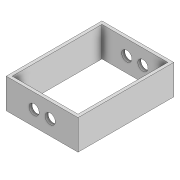
# Autodesk Inventor part: 본체 겉면
Saved by Autodesk Inventor 2020 (Build 240168000, 168)
## iProperties
Created: 2022-08-24
Part Number: 본체 겉면
Material: 일반
Document SubType Name: Modeling
Designer: 박연호
Density: 1 g/cm^3
Appearance: 기본값
Author: 박연호
Autodesk Inventor part; units mm, degrees
ref_plane "YZ Plane" through (0, 0, 0) normal (1, 0, 0) x (0, 1, 0)
ref_plane "XZ Plane" through (0, 0, 0) normal (0, 1, 0) x (-1, 0, 0)
ref_plane "XY Plane" through (0, 0, 0) normal (0, 0, 1) x (1, 0, 0)
sketch "스케치1" plane through (0, 0, 0) normal (0, 1, 0) x (-1, 0, 0)
  line L0 (60, 80) -> (-60, 80)
  line L1 (-60, 80) -> (-60, -80)
  line L2 (-60, -80) -> (60, -80)
  line L3 (60, -80) -> (60, 80)
  line L4 (60, 80) -> (-60, -80) construction
  line L5 (-60, 80) -> (60, -80) construction
  point P0 (0, 0)
  dimension "d0" = 120
  dimension "d1" = 160
  constraints: 12 end point, 2 midpoint, 2 parallel, 1 horizontal, 1 perpendicular
  measures "d0" distance of L0.start L0.end
  measures "d1" distance of L0.end L1.end
extrude "돌출1" add sketch "스케치1" along normal blind 60
sketch "스케치2" plane through (0, 60, 0) normal (0, 1, 0) x (1, 0, 0)
  line L0 (60, -80) -> (60, 80) projected
  line L1 (60, 80) -> (-60, 80) projected
  line L2 (55, 102.1646) -> (-55, 102.1646)
  line L3 (-55, 102.1646) -> (-55, -89.711)
  line L4 (-55, -89.711) -> (55, -89.711)
  line L5 (55, -89.711) -> (55, 102.1646)
  line L6 (-60, 80) -> (-60, -80) projected
  point P0 (0, 0)
  point P1 (55, 80)
  point P2 (-55, 80)
  dimension "d6" = 5
  dimension "d7" = 5
  constraints: 8 end point, 2 parallel, 1 horizontal, 1 perpendicular
  measures "d6" distance between parallel lines of L5 L0
  measures "d7" distance between parallel lines of L6 L3
extrude "돌출2" cut sketch "스케치2" against normal blind 40 contours L5 L4 L3 L1
sketch "스케치12" plane through (60, 0, -80) normal (0, 0, -1) x (-1, 0, 0)
  line L0 (-34.8463, 10) -> (156.2634, 10)
  line L1 (156.2634, 10) -> (156.2634, -36.9465)
  line L2 (156.2634, -36.9465) -> (-34.8463, -36.9465)
  line L3 (-34.8463, -36.9465) -> (-34.8463, 10)
  line L4 (0, 0) -> (120, 0) projected
  point P0 (60, 0)
  dimension "d85" = 10
  constraints: 8 end point, 2 parallel, 1 horizontal, 1 perpendicular
  measures "d85" distance between parallel lines of L4 L0
extrude "돌출10" cut sketch "스케치12" against normal through all
sketch "스케치13" plane through (-55, 20, 80) normal (0, 0, 1) x (1, 0, 0)
  line L0 (0, 40) -> (0, 0) projected
  line L1 (0, 0) -> (110, 0) projected
  line L2 (0, 40) -> (110, 40)
  line L3 (110, 40) -> (110, 0)
  line L4 (110, 0) -> (0, 0)
  line L5 (0, 0) -> (0, 40)
  point P0 (55, -20)
  constraints: 8 end point, 2 parallel, 1 horizontal, 1 perpendicular
extrude "돌출11" add sketch "스케치13" against normal blind 5
sketch "스케치14" plane through (55, 20, -80) normal (0, 0, -1) x (-1, 0, 0)
  line L0 (0, 0) -> (0, 40) projected
  line L1 (110, 0) -> (0, 0) projected
  line L2 (0, 40) -> (110, 40)
  line L3 (110, 40) -> (110, 0)
  line L4 (110, 0) -> (0, 0)
  line L5 (0, 0) -> (0, 40)
  point P0 (55, -20)
  constraints: 8 end point, 2 parallel, 1 horizontal, 1 perpendicular
extrude "돌출12" add sketch "스케치14" against normal blind 5
sketch "스케치15" plane through (60, 60, -80) normal (0, 0, -1) x (-1, 0, 0)
  point P0 (60, -60)
sketch "스케치16" plane through (60, 60, -80) normal (0, 0, -1) x (-1, 0, 0)
  point P0 (60, -60)
sketch "스케치17" plane through (0, 20, 0) normal (0, 1, 0) x (1, 0, 0)
  line L0 (7, 27) -> (45, 27)
  line L1 (45, 27) -> (45, 65)
  line L2 (45, 65) -> (7, 65)
  line L3 (7, 65) -> (7, 27)
  line L4 (55, 75) -> (55, -75) projected
  line L5 (55, 75) -> (-55, 75) projected
  circle A0 centre (7, 27) radius 1.6
  circle A1 centre (7, 65) radius 1.6
  circle A2 centre (45, 65) radius 1.6
  circle A3 centre (45, 27) radius 1.6
  line L6 (-47.9371, 14.7215) -> (-7.9371, 14.7215)
  line L7 (-7.9371, 14.7215) -> (-7.9371, 64.7215)
  line L8 (-7.9371, 64.7215) -> (-47.9371, 64.7215)
  line L9 (-47.9371, 64.7215) -> (-47.9371, 14.7215)
  point P0 (0, 0)
  dimension "d92" = 38
  dimension "d93" = 38
  dimension "d95" = 10
  dimension "d96" = 10
  dimension "d97" = 3.2
  dimension "d98" = 3.2
  dimension "d99" = 3.2
  dimension "d100" = 3.2
  dimension "d113" = 40
  dimension "d114" = 50
  constraints: 16 end point, 4 centre point, 4 coincident, 4 parallel, 2 horizontal, 2 perpendicular
  measures "d92" distance of L2.end L0.start
  measures "d93" distance of L1.end L2.end
  measures "d95" distance between parallel lines of L4 L1
  measures "d96" distance between parallel lines of L5 L2
  measures "d97" diameter of A0
  measures "d98" diameter of A1
  measures "d99" diameter of A2
  measures "d100" diameter of A3
  measures "d113" distance of L7.end L8.end
  measures "d114" distance of L8.end L6.start
extrude "돌출13" cut sketch "스케치17" against normal through all contours L3 A0 L0 | L0 A0 L3 | A3 L1 L0 | L0 L1 A3 | A1 L2 L3 | L3 L2 A1 | A2 L2 L1 | L1 L2 A2
sketch "스케치19" plane through (60, 60, -80) normal (0, 0, -1) x (-1, 0, 0)
  line L0 (5, -40) -> (115, -40) projected
  circle A0 centre (46.5, -25) radius 8.5
  circle A1 centre (73.5, -25) radius 8.5
  line L1 (5, 0) -> (5, -40) projected
  line L2 (115, -40) -> (115, 0) projected
  point P0 (60, -60)
  dimension "d105" = 27
  dimension "d106" = 41.5
  dimension "d107" = 17
  dimension "d108" = 17
  dimension "d109" = 15
  dimension "d110" = 15
  constraints: 2 centre point
  measures "d105" distance of A1.centre A0.centre
  measures "d106" distance from line of L1 A0.centre
  measures "d107" diameter of A0
  measures "d108" diameter of A1
  measures "d109" distance from line of L0 A1.centre
  measures "d110" distance from line of L0 A0.centre
extrude "돌출14" cut sketch "스케치19" against normal through all
sketch "스케치21" plane through (0, 20, 0) normal (0, 1, 0) x (1, 0, 0)
  circle A0 centre (5.4243, 8.1678) radius 7.5
  line L0 (-49.3888, 17.2731) -> (-9.3888, 17.2731)
  line L1 (-9.3888, 17.2731) -> (-9.3888, 67.2731)
  line L2 (-9.3888, 67.2731) -> (-49.3888, 67.2731)
  line L3 (-49.3888, 67.2731) -> (-49.3888, 17.2731)
  point P0 (0, 0)
  dimension "d117" = 15
  dimension "d118" = 50
  dimension "d119" = 40
  constraints: 8 end point, 2 parallel, 1 centre point, 1 horizontal, 1 perpendicular
  measures "d117" diameter of A0
  measures "d118" distance of L2.end L0.start
  measures "d119" distance of L1.end L2.end
extrude "돌출15" cut sketch "스케치21" against normal through all contours A0
sketch "스케치23" plane through (0, 20, 0) normal (0, 1, 0) x (1, 0, 0)
  line L0 (-48.6, -65) -> (20, -65)
  line L1 (20, -65) -> (20, -11.6)
  line L2 (20, -11.6) -> (-48.6, -11.6)
  line L3 (-48.6, -11.6) -> (-48.6, -65)
  line L4 (55, 75) -> (55, -75) projected
  line L5 (-55, -75) -> (55, -75) projected
  circle A0 centre (4.7, -62.45) radius 1.6
  circle A1 centre (6.03, -14.15) radius 1.6
  circle A2 centre (-46.05, -47.16) radius 1.6
  circle A3 centre (-46.05, -19.23) radius 1.6
  point P0 (0, 0)
  dimension "d123" = 68.6
  dimension "d124" = 53.4
  dimension "d125" = 35
  dimension "d126" = 10
  dimension "d127" = 3.2
  dimension "d128" = 15.3
  dimension "d129" = 2.55
  dimension "d130" = 3.2
  dimension "d131" = 13.97
  dimension "d132" = 2.55
  dimension "d133" = 3.2
  dimension "d134" = 35.56
  dimension "d135" = 3.2
  dimension "d136" = 2.55
  dimension "d137" = 2.55
  dimension "d138" = 7.63
  constraints: 8 end point, 4 centre point, 2 parallel, 1 horizontal, 1 perpendicular
  measures "d123" distance of L1.end L2.end
  measures "d124" distance of L2.end L0.start
  measures "d125" distance between parallel lines of L4 L1
  measures "d126" distance between parallel lines of L5 L0
  measures "d127" diameter of A0
  measures "d128" distance from line of L1 A0.centre
  measures "d129" distance from line of A0.centre L0
  measures "d130" diameter of A1
  measures "d131" distance from line of L1 A1.centre
  measures "d132" distance from line of L2 A1.centre
  measures "d133" diameter of A2
  measures "d134" distance from line of L2 A2.centre
  measures "d135" diameter of A3
  measures "d136" distance from line of L3 A3.centre
  measures "d137" distance from line of L3 A2.centre
  measures "d138" distance from line of L2 A3.centre
extrude "돌출16" cut sketch "스케치23" against normal through all contours A0 | A1 | A2 | A3
sketch "스케치24" plane through (0, 20, 0) normal (0, 1, 0) x (1, 0, 0)
  line L0 (-55, -75) -> (55, -75) projected
  line L1 (55, 75) -> (55, -75) projected
  line L2 (-55, -75) -> (55, -75)
  line L3 (55, -75) -> (55, 75)
  line L4 (55, 75) -> (-55, 75)
  line L5 (-55, 75) -> (-55, -75)
  point P0 (0, 0)
  constraints: 8 end point, 2 parallel, 1 horizontal, 1 perpendicular
extrude "돌출17" cut sketch "스케치24" against normal through all
